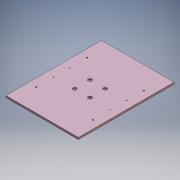
# Autodesk Inventor part: piStagesAttach
Saved by Autodesk Inventor 2016 (Build 200138000, 138)
## iProperties
Created: 2016-03-15
Part Number: piStagesAttach
Material: Generic
Document SubType Name: Modeling
Designer: sims01
Density: 1 g/cm^3
Appearance: Default
Author: sims01
Autodesk Inventor part; units mm, degrees
ref_plane "YZ Plane" through (0, 0, 0) normal (1, 0, 0) x (0, 1, 0)
ref_plane "XZ Plane" through (0, 0, 0) normal (0, 1, 0) x (-1, 0, 0)
ref_plane "XY Plane" through (0, 0, 0) normal (0, 0, 1) x (1, 0, 0)
sketch "Sketch1" plane through (0, 0, 0) normal (0, 0, 1) x (1, 0, 0)
  line L0 (-148, 200) -> (148, 200)
  line L1 (148, 200) -> (148, -200)
  line L2 (148, -200) -> (-148, -200)
  line L3 (-148, -200) -> (-148, 200)
  point P0 (0, 0)
  dimension "d0" = 400
  dimension "d1" = 296
  dimension "d2" = 148
  dimension "d3" = 200
  constraints: 8 end point, 2 parallel, 1 horizontal, 1 perpendicular
  measures "d0" distance of L0.end L1.end
  measures "d1" distance of L0.start L0.end
  measures "d2" distance from line of point (0, 0) L1
  measures "d3" distance from line of point (0, 0) L0
extrude "baseExtrusion" add sketch "Sketch1" along normal blind 10
sketch "Sketch2" plane through (0, 0, 10) normal (0, 0, 1) x (1, 0, 0)
  line L0 (-148, 200) -> (-148, -200) projected
  line L1 (148, -200) -> (148, 200) projected
  line L2 (148, 200) -> (-148, 200) projected
  point P0 (0, 0)
  point P1 (-139.5, 40)
  point P2 (139.5, 40)
  point P3 (-139.5, -40)
  point P4 (139.5, -40)
  dimension "d6" = 8.5
  dimension "d7" = 8.5
  dimension "d22" = 160
  dimension "d23" = 240
  constraints: 2 horizontal alignment, 2 vertical alignment
  measures "d6" distance from line of L0 point (-139.5, 40)
  measures "d7" distance from line of L1 point (139.5, 40)
  measures "d22" distance from line of point (-139.5, 40) L2
  measures "d23" distance from line of point (-139.5, -40) L2
hole "xyStageAttach_m5" at (-139.5, 40, 10) at (139.5, 40, 10) at (-139.5, -40, 10) at (139.5, -40, 10) direction (0, 0, -1) diameter 4.134 depth 14.2 tip angle 118 thread size "M5x0.8" class "6H" standard "ISO Metric profile"
sketch "Sketch4" plane through (0, 0, 10) normal (0, 0, 1) x (1, 0, 0)
  point P0 (0, 0)
  point P1 (-37.5, 37.5)
  point P2 (37.5, 37.5)
  point P3 (-37.5, -37.5)
  point P4 (37.5, -37.5)
  dimension "d24" = 75
  dimension "d25" = 75
  dimension "d26" = 37.5
  dimension "d27" = 37.5
  constraints: 2 horizontal alignment, 2 vertical alignment
  measures "d24" distance of point (37.5, 37.5) point (-37.5, 37.5)
  measures "d25" distance of point (37.5, -37.5) point (37.5, 37.5)
  measures "d26" horizontal distance of point (0, 0) point (37.5, 37.5)
  measures "d27" horizontal distance of point (0, 0) point (37.5, 37.5)
hole "zStageAttach_m6" at (-37.5, 37.5, 10) at (37.5, 37.5, 10) at (-37.5, -37.5, 10) at (37.5, -37.5, 10) direction (0, 0, -1) diameter 6.6 depth 17.1 tip angle 118 counterbore diameter 18 counterbore depth 4.8 clearance for "Hex Head Cap Screw ISO 24017" size "M6" standard "ISO"
sketch "Sketch5" plane through (0, 0, 10) normal (0, 0, 1) x (1, 0, 0)
  line L0 (-178, 235) -> (178, 235)
  line L1 (178, 235) -> (178, -235)
  line L2 (178, -235) -> (-178, -235)
  line L3 (-178, -235) -> (-178, 235)
  line L4 (-148, 200) -> (-148, -200) projected
  line L5 (148, -200) -> (148, 200) projected
  line L6 (148, 200) -> (-148, 200) projected
  line L7 (-148, -200) -> (148, -200) projected
  point P0 (0, 0)
  dimension "d35" = 30
  dimension "d36" = 30
  dimension "d37" = 35
  dimension "d38" = 35
  constraints: 8 end point, 2 parallel, 1 horizontal, 1 perpendicular
  measures "d35" distance between parallel lines of L3 L4
  measures "d36" distance between parallel lines of L1 L5
  measures "d37" distance between parallel lines of L0 L6
  measures "d38" distance between parallel lines of L2 L7
extrude "attachmentExtrusion" add sketch "Sketch5" against normal blind 10
sketch "Sketch9" plane through (0, 0, 0) normal (0, 0, -1) x (-1, 0, 0)
  point P0 (0, 0)
  point P1 (-139.5, 125)
  point P2 (139.5, 125)
  point P3 (-139.5, -125)
  point P4 (139.5, -125)
  dimension "d67" = 250
  dimension "d69" = 279
  dimension "d70" = 139.5
  dimension "d78" = 125
  constraints: 2 horizontal alignment, 2 vertical alignment
  measures "d67" distance of point (-139.5, -125) point (-139.5, 125)
  measures "d69" distance of point (139.5, 125) point (-139.5, 125)
  measures "d70" horizontal distance of point (0, 0) point (-139.5, 125)
  measures "d78" vertical distance of point (0, 0) point (-139.5, 125)
hole "postAttach_m6" at (139.5, 125, 0) at (-139.5, 125, 0) at (139.5, -125, 0) at (-139.5, -125, 0) direction (0, 0, 1) diameter 6.6 depth 17.1 tip angle 118 counterbore diameter 18 counterbore depth 4.8 clearance for "Hex Head Cap Screw ISO 24017" size "M6" standard "ISO"
equation "\"d2\" = 0.5 * d1"
equation "\"d3\" = 0.5 * d0"
equation "\"d7\" = d6"
equation "\"d26\" = 0.5 * d24"
equation "\"d27\" = 0.5 * d25"
equation "\"d36\" = d35"
equation "\"d38\" = d37"
equation "\"d70\" = 0.5 * d69"
equation "\"d78\" = 0.5 * d67"
body "Solid1"
